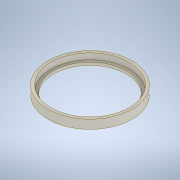
# Autodesk Inventor part: внешнее кольцо подшипника
Saved by Autodesk Inventor 2020.1 (Build 241239000, 239)
## iProperties
Created: 2022-04-01
Part Number: внешнее кольцо подшипника
Material: Титан
Document SubType Name: Modeling
Designer: User
Density: 4.51 g/cm^3
Appearance: Титан
Author: User
Autodesk Inventor part; units mm, degrees
ref_plane "YZ Plane" through (0, 0, 0) normal (1, 0, 0) x (0, 1, 0)
ref_plane "XZ Plane" through (0, 0, 0) normal (0, 1, 0) x (-1, 0, 0)
ref_plane "XY Plane" through (0, 0, 0) normal (0, 0, 1) x (1, 0, 0)
sketch "Эскиз1" plane through (0, 0, 0) normal (0, 1, 0) x (-1, 0, 0)
  circle A0 centre (0, 0) radius 60
  circle A1 centre (0, 0) radius 52
  point P0 (0, 52)
  point P1 (0, 60)
  dimension "d0" = 120
  dimension "d3" = 8
  constraints: 2 coincident, 2 vertical alignment, 4 other
  measures "d3" distance of point (0, 60) point (0, 52)
extrude "Выдавливание1" add sketch "Эскиз1" along normal blind 4
sketch "Эскиз2" plane through (0, 4, 0) normal (0, 1, 0) x (1, 0, 0)
  circle A0 centre (0, 0) radius 60
  circle A1 centre (0, 0) radius 56
  circle A2 centre (0, 0) radius 60 projected
  point P0 (0, -56)
  point P1 (0, -60)
  point P2 (0, -60)
  dimension "d4" = 4
  dimension "d5" = 0
  constraints: 3 vertical alignment, 2 coincident, 5 other
  measures "d4" distance of point (0, -56) point (0, -60)
  measures "d5" distance of point (0, -60) point (0, -60)
extrude "Выдавливание2" add sketch "Эскиз2" along normal blind 8.5
